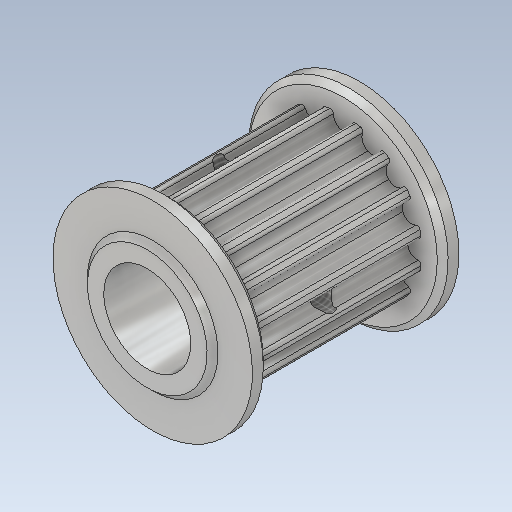
# Autodesk Inventor part: Motor Pulley
Saved by Autodesk Inventor 2020.1 (Build 241239000, 239)
## iProperties
Created: 2018-11-27
Part Number: Motor Pulley
Material: Aluminum 6061-AHC
Document SubType Name: Modeling
Designer: Petar
Density: 2.7 g/cm^3
Appearance: Aluminum - Dark
Mass: 5.37711 g
Surface Area: 24.7132 cm^2
Volume: 1.99152 cm^3
Author: Petar
Autodesk Inventor part; units mm, degrees
ref_plane "YZ Plane" through (0, 0, 0) normal (1, 0, 0) x (0, 1, 0)
derived "gates_P16-3M-09AL.ipt"
sketch "Sketch1" plane through (0, 0, 0) normal (0, 0, -1) x (-1, 0, 0)
  circle A0 centre (0, 0) radius 8.1407
  arc A1 (1.6488, 7.0748) -> (1.203, 7.1641) centre (0, 0) ccw
  arc A2 (1.8152, 6.7077) -> (1.6488, 7.0748) centre (1.5912, 6.8274) ccw
  arc A3 (1.8152, 6.7077) -> (2.2747, 5.4917) centre (2.5768, 6.3007) ccw
  arc A4 (2.2747, 5.4917) -> (3.4596, 6.0266) centre (2.5976, 6.3562) ccw
  arc A5 (3.853, 6.1584) -> (3.4596, 6.0266) centre (3.7105, 5.9306) ccw
  arc A6 (4.2307, 5.9053) -> (3.853, 6.1584) centre (0, 0) ccw
  arc A7 (4.2439, 5.5025) -> (4.2307, 5.9053) centre (4.0828, 5.6988) ccw
  arc A8 (4.2439, 5.5025) -> (4.2031, 4.2031) centre (4.7919, 4.835) ccw
  arc A9 (4.2031, 4.2031) -> (5.5025, 4.2439) centre (4.8323, 4.8783) ccw
  arc A10 (5.9164, 4.2152) -> (5.5025, 4.2439) centre (5.6976, 4.0593) ccw
  arc A11 (6.1685, 3.8368) -> (5.9164, 4.2152) centre (0, 0) ccw
  arc A12 (6.0266, 3.4596) -> (6.1685, 3.8368) centre (5.9528, 3.7026) ccw
  arc A13 (6.0266, 3.4596) -> (5.4917, 2.2747) centre (6.2774, 2.6332) ccw
  arc A14 (5.4917, 2.2747) -> (6.7077, 1.8152) centre (6.3313, 2.6578) ccw
  arc A15 (7.0791, 1.6302) -> (6.7077, 1.8152) centre (6.8173, 1.5699) ccw
  arc A16 (7.1672, 1.1841) -> (7.0791, 1.6302) centre (0, 0) ccw
  arc A17 (6.8918, 0.8899) -> (7.1672, 1.1841) centre (6.9166, 1.1427) ccw
  arc A18 (6.8918, 0.8899) -> (5.9441, 0) centre (6.8072, 0.0305) ccw
  arc A19 (5.9441, 0) -> (6.8918, -0.8899) centre (6.8664, 0.0326) ccw
  arc A20 (7.1641, -1.203) -> (6.8918, -0.8899) centre (6.8991, -1.1585) ccw
  arc A21 (7.0748, -1.6488) -> (7.1641, -1.203) centre (0, 0) ccw
  arc A22 (6.7077, -1.8152) -> (7.0748, -1.6488) centre (6.8274, -1.5912) ccw
  arc A23 (6.7077, -1.8152) -> (5.4917, -2.2747) centre (6.3007, -2.5768) ccw
  arc A24 (5.4917, -2.2747) -> (6.0266, -3.4596) centre (6.3562, -2.5976) ccw
  arc A25 (6.1584, -3.853) -> (6.0266, -3.4596) centre (5.9306, -3.7105) ccw
  arc A26 (5.9053, -4.2307) -> (6.1584, -3.853) centre (0, 0) ccw
  arc A27 (5.5025, -4.2439) -> (5.9053, -4.2307) centre (5.6988, -4.0828) ccw
  arc A28 (5.5025, -4.2439) -> (4.2031, -4.2031) centre (4.835, -4.7919) ccw
  arc A29 (4.2031, -4.2031) -> (4.2439, -5.5025) centre (4.8783, -4.8323) ccw
  arc A30 (4.2152, -5.9164) -> (4.2439, -5.5025) centre (4.0593, -5.6976) ccw
  arc A31 (3.8368, -6.1685) -> (4.2152, -5.9164) centre (0, 0) ccw
  arc A32 (3.4596, -6.0266) -> (3.8368, -6.1685) centre (3.7026, -5.9528) ccw
  arc A33 (3.4596, -6.0266) -> (2.2747, -5.4917) centre (2.6332, -6.2774) ccw
  arc A34 (2.2747, -5.4917) -> (1.8152, -6.7077) centre (2.6578, -6.3313) ccw
  arc A35 (1.6302, -7.0791) -> (1.8152, -6.7077) centre (1.5699, -6.8173) ccw
  arc A36 (1.1841, -7.1672) -> (1.6302, -7.0791) centre (0, 0) ccw
  arc A37 (0.8899, -6.8918) -> (1.1841, -7.1672) centre (1.1427, -6.9166) ccw
  arc A38 (0.8899, -6.8918) -> (0, -5.9441) centre (0.0305, -6.8072) ccw
  arc A39 (0, -5.9441) -> (-0.8899, -6.8918) centre (0.0326, -6.8664) ccw
  arc A40 (-1.203, -7.1641) -> (-0.8899, -6.8918) centre (-1.1585, -6.8991) ccw
  arc A41 (-1.6488, -7.0748) -> (-1.203, -7.1641) centre (0, 0) ccw
  arc A42 (-1.8152, -6.7077) -> (-1.6488, -7.0748) centre (-1.5912, -6.8274) ccw
  arc A43 (-1.8152, -6.7077) -> (-2.2747, -5.4917) centre (-2.5768, -6.3007) ccw
  arc A44 (-2.2747, -5.4917) -> (-3.4596, -6.0266) centre (-2.5976, -6.3562) ccw
  arc A45 (-3.853, -6.1584) -> (-3.4596, -6.0266) centre (-3.7105, -5.9306) ccw
  arc A46 (-4.2307, -5.9053) -> (-3.853, -6.1584) centre (0, 0) ccw
  arc A47 (-4.2439, -5.5025) -> (-4.2307, -5.9053) centre (-4.0828, -5.6988) ccw
  arc A48 (-4.2439, -5.5025) -> (-4.2031, -4.2031) centre (-4.7919, -4.835) ccw
  arc A49 (-4.2031, -4.2031) -> (-5.5025, -4.2439) centre (-4.8323, -4.8783) ccw
  arc A50 (-5.9164, -4.2152) -> (-5.5025, -4.2439) centre (-5.6976, -4.0593) ccw
  arc A51 (-6.1685, -3.8368) -> (-5.9164, -4.2152) centre (0, 0) ccw
  arc A52 (-6.0266, -3.4596) -> (-6.1685, -3.8368) centre (-5.9528, -3.7026) ccw
  arc A53 (-6.0266, -3.4596) -> (-5.4917, -2.2747) centre (-6.2774, -2.6332) ccw
  arc A54 (-5.4917, -2.2747) -> (-6.7077, -1.8152) centre (-6.3313, -2.6578) ccw
  arc A55 (-7.0791, -1.6302) -> (-6.7077, -1.8152) centre (-6.8173, -1.5699) ccw
  arc A56 (-7.1672, -1.1841) -> (-7.0791, -1.6302) centre (0, 0) ccw
  arc A57 (-6.8918, -0.8899) -> (-7.1672, -1.1841) centre (-6.9166, -1.1427) ccw
  arc A58 (-6.8918, -0.8899) -> (-5.9441, 0) centre (-6.8072, -0.0305) ccw
  arc A59 (-5.9441, 0) -> (-6.8918, 0.8899) centre (-6.8664, -0.0326) ccw
  arc A60 (-7.1641, 1.203) -> (-6.8918, 0.8899) centre (-6.8991, 1.1585) ccw
  arc A61 (-7.0748, 1.6488) -> (-7.1641, 1.203) centre (0, 0) ccw
  arc A62 (-6.7077, 1.8152) -> (-7.0748, 1.6488) centre (-6.8274, 1.5912) ccw
  arc A63 (-6.7077, 1.8152) -> (-5.4917, 2.2747) centre (-6.3007, 2.5768) ccw
  arc A64 (-5.4917, 2.2747) -> (-6.0266, 3.4596) centre (-6.3562, 2.5976) ccw
  arc A65 (-6.1584, 3.853) -> (-6.0266, 3.4596) centre (-5.9306, 3.7105) ccw
  arc A66 (-5.9053, 4.2307) -> (-6.1584, 3.853) centre (0, 0) ccw
  arc A67 (-5.5025, 4.2439) -> (-5.9053, 4.2307) centre (-5.6988, 4.0828) ccw
  arc A68 (-5.5025, 4.2439) -> (-4.2031, 4.2031) centre (-4.835, 4.7919) ccw
  arc A69 (-4.2031, 4.2031) -> (-4.2439, 5.5025) centre (-4.8783, 4.8323) ccw
  arc A70 (-4.2152, 5.9164) -> (-4.2439, 5.5025) centre (-4.0593, 5.6976) ccw
  arc A71 (-3.8368, 6.1685) -> (-4.2152, 5.9164) centre (0, 0) ccw
  arc A72 (-3.4596, 6.0266) -> (-3.8368, 6.1685) centre (-3.7026, 5.9528) ccw
  arc A73 (-3.4596, 6.0266) -> (-2.2747, 5.4917) centre (-2.6332, 6.2774) ccw
  arc A74 (-2.2747, 5.4917) -> (-1.8152, 6.7077) centre (-2.6578, 6.3313) ccw
  arc A75 (-1.6302, 7.0791) -> (-1.8152, 6.7077) centre (-1.5699, 6.8173) ccw
  arc A76 (-1.1841, 7.1672) -> (-1.6302, 7.0791) centre (0, 0) ccw
  arc A77 (-0.8899, 6.8918) -> (-1.1841, 7.1672) centre (-1.1427, 6.9166) ccw
  arc A78 (-0.8899, 6.8918) -> (0, 5.9441) centre (-0.0305, 6.8072) ccw
  arc A79 (0, 5.9441) -> (0.8899, 6.8918) centre (-0.0326, 6.8664) ccw
  arc A80 (1.203, 7.1641) -> (0.8899, 6.8918) centre (1.1585, 6.8991) ccw
extrude "Extrusion7" add sketch "Sketch1" along normal blind 16 contours A2 A3 A4 A5 A6 A7 A8 A9 A10 A11 A12 A13 A14 A15 A16 A17 A18 A19 A20 A21 A22 A23 A24 A25 A26 A27 A28 A29 A30 A31 A32 A33 A34 A35 A36 A37 A38 A39 A40 A41 A42 A43 A44 A45 A46 A47 A48 A49 A50 A51 A52 A53 A54 A55 A56 A57 A58 A59 A60 A61 A62 A63 A64 A65 A66 A67 A68 A69 A70 A71 A72 A73 A74 A75 A76 A77 A78 A79 A80 A1
sketch "Sketch14" plane through (-2.5768, 6.3007, 0) normal (0, 0, 1) x (0.935435, -0.3534987, 0)
  circle A0 centre (4.6378, -4.983) radius 4
  dimension "d54" = 8
  constraints: 1 centre point, 1 coincident
  measures "d54" diameter of A0
extrude "Extrusion8" cut sketch "Sketch14" against normal through all
sketch "Sketch15" plane through (0, 0, 0) normal (1, 0, 0) x (0, 1, 0)
  line L0 (9.1672, 1.5) -> (9.1672, 0)
  line L1 (9.1672, 0) -> (4, 0)
  line L2 (4, 0) -> (4, 2)
  line L3 (7.1672, 0) -> (7.1672, -16) construction
  line L4 (-4, 0) -> (4, 0) construction
  line L5 (6, 1.5) -> (6, 2)
  line L6 (6, 2) -> (4, 2)
  line L7 (6, 1.5) -> (9.1672, 1.5)
  line L8 (0, 6.8) -> (0, -19.8) projected
  point P0 (0, 0)
  dimension "d57" = 2
  dimension "d58" = 1.5
  dimension "d59" = 2
  dimension "d60" = 0.5
  constraints: 12 end point, 3 parallel, 2 point on line, 1 horizontal, 1 perpendicular
  measures "d57" distance between parallel lines of L0 L3
  measures "d58" distance of L0.start L0.end
  measures "d59" distance of L2.end L5.end
  measures "d60" distance of L5.start L5.end
revolve "Revolution2" add sketch "Sketch15" angle 360 about axis through (0, 0, 0) along (0, 0, -1)
chamfer "Chamfer2" distance 0.5 angle 45 2 edges at (0, -9.1672, 0) (0, -6, 2)
ref_plane "Work Plane3" through (0.0305, 6.8072, -8) normal (0, 0, -1) x (-0.7289512, 0.6845657, 0)
mirror "Mirror1" about plane through (0.0305, 6.8072, -8) normal (0, 0, -1) of "Revolution2", "Chamfer2"
ref_plane "Work Plane4" through (-5.9053, -4.2307, 0) normal (-0.7061752, -0.7080371, 0) x (0, 0, -1)
sketch "Sketch16" plane through (-5.9053, -4.2307, 0) normal (-0.7061752, -0.7080371, 0) x (0, 0, -1)
  line L0 (0, 1.2014) -> (16, 1.2014) construction
  circle A0 centre (8, 1.2014) radius 1
  point P0 (0, 1.1935)
  dimension "d65" = 2
  constraints: 1 centre point, 2 other
  measures "d65" diameter of A0
extrude "Extrusion9" cut sketch "Sketch16" against normal up to surface round surface about axis through (0, 0, 0) along (0, 0, -1) radius 4 far side no
thread "Thread2" size "M2x0.4" class "6H" standard "ANSI Metric M Profile" full length
pattern_circular "Circular Pattern1" count 2 over 112.45 about axis through (0, 0, 0) along (0, 0, -1) of "Extrusion9"
pattern_circular "Circular Pattern2" count 2 over 135 about axis through (0, 0, 0) along (0, 0, 1) of "Extrusion9"
body "Solid3"
